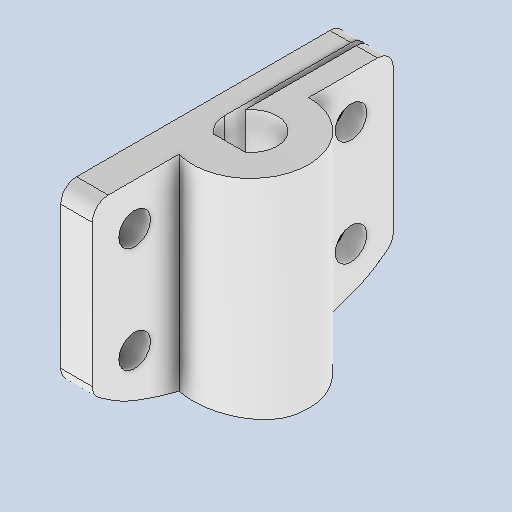
# Autodesk Inventor part: eixo_motor
Saved by Autodesk Inventor 2023.2 (Build 272271000, 271)
## iProperties
Created: 2023-04-13
Part Number: eixo_motor
Material: ABS plástico
Document SubType Name: Modeling
Designer: Edilson
Density: 1.06 g/cm^3
Appearance: Suave - Branco
Author: Edilson
Autodesk Inventor part; units mm, degrees
ref_plane "YZ Plane" through (0, 0, 0) normal (1, 0, 0) x (0, 1, 0)
ref_plane "XZ Plane" through (0, 0, 0) normal (0, 1, 0) x (-1, 0, 0)
sketch "Esboço5" plane through (0, 0, 0) normal (0, 1, 0) x (-1, 0, 0)
  line L0 (-13.5, 0) -> (-13.5, -1)
  line L1 (-13.5, -1) -> (0, -1)
  line L2 (13.5, -1) -> (13.5, 0)
  arc A0 (-5.5, -3.5) -> (5.2915, -2) centre (0, -3.5) ccw
  line L3 (2, -3.5) -> (2, -2)
  line L4 (2, -3.5) -> (2, -5)
  line L5 (-13.5, -1.5) -> (-1.5, -1.5)
  line L6 (-13.5, -1.5) -> (-13.5, -3.5)
  line L7 (-13.5, -3.5) -> (-5.5, -3.5)
  line L8 (13.5, -1) -> (13.5, -2)
  line L9 (13.5, -2) -> (5.2915, -2)
  arc A1 (2, -2) -> (0, -1) centre (0, -3.5) ccw
  arc A2 (-1.5, -1.5) -> (2, -5) centre (0, -3.5) ccw
  line L10 (13.5, 0) -> (13.5, 1)
  line L11 (13.5, 0) -> (14.5, 0) construction
  line L12 (13.5, 1) -> (-13.5, 1)
  line L13 (-13.5, 1) -> (-13.5, 0)
  constraints: 28 end point, 6 perpendicular, 6 point on circle, 3 centre point, 1 horizontal, 1 parallel, 1 point on line, 1 vertical
extrude "Extrusão4" add sketch "Esboço5" against normal blind 20
sketch "Esboço6" plane through (-5.2915, 0, -2) normal (0, 0, -1) x (-1, 0, 0)
  circle A0 centre (4.2085, -16) radius 1.5
  circle A1 centre (4.2085, -6) radius 1.5
  line L0 (8.2085, -20) -> (0, -20) projected
  line L1 (8.2085, 0) -> (8.2085, -20) projected
  point P0 (-5.2915, 0)
  point P1 (4.1042, -20)
  dimension "d51" = 3
  dimension "d52" = 3
  dimension "d53" = 4
  dimension "d54" = 4
  dimension "d55" = 10
  dimension "d56" = 4
  constraints: 2 centre point, 1 midpoint
  measures "d51" diameter of A0
  measures "d52" diameter of A1
  measures "d53" vertical distance of point (4.104, -20) A0.centre
  measures "d54" distance from line of L1 A0.centre
  measures "d55" distance of A1.centre A0.centre
  measures "d56" distance from line of L1 A1.centre
extrude "Extrusão5" cut sketch "Esboço6" against normal through all
sketch "Esboço7" plane through (13.5, 0, -3.5) normal (0, 0, -1) x (-1, 0, 0)
  circle A0 centre (4, -16) radius 1.5
  circle A1 centre (4, -6) radius 1.5
  line L0 (8, -20) -> (0, -20) projected
  line L1 (0, 0) -> (0, -20) projected
  point P0 (13.5, 0)
  point P1 (4, -20)
  dimension "d59" = 3
  dimension "d60" = 3
  dimension "d61" = 4
  dimension "d62" = 4
  dimension "d63" = 4
  dimension "d64" = 10
  constraints: 2 centre point, 1 midpoint
  measures "d59" diameter of A0
  measures "d60" diameter of A1
  measures "d61" distance of point (4, -20) A0.centre
  measures "d62" distance from line of L1 A0.centre
  measures "d63" distance from line of L1 A1.centre
  measures "d64" distance of A1.centre A0.centre
extrude "Extrusão6" cut sketch "Esboço7" against normal through all
ref_plane "Plano de trabalho2" through (-12, 0, 1) normal (0, 0, 1) x (1, 0, 0)
sketch "Esboço9" plane through (-12, 0, 1) normal (0, 0, 1) x (1, 0, 0)
  spline S0 degree 3 poles (57.7409, -54.8608) (52.9733, -36.0784) (42.5201, -20.9336) (27.3088, -10.4014) knots 0 0 0 0 1 1 1 1
  line L0 (57.7409, -54.8608) -> (52.9733, -36.0784) construction
  line L1 (52.9733, -36.0784) -> (42.5201, -20.9336) construction
  line L2 (42.5201, -20.9336) -> (27.3088, -10.4014) construction
  line L3 (27.3088, -10.4014) -> (21.7838, -6.5759)
  spline S1 degree 3 poles (21.7838, -6.5759) (20.7493, -5.8596) (20.3116, -5.8348) (19.1032, -5.4031) knots 0 0 0 0 1 1 1 1
  line L4 (21.7838, -6.5759) -> (20.7493, -5.8596) construction
  line L5 (20.7493, -5.8596) -> (20.3116, -5.8348) construction
  line L6 (20.3116, -5.8348) -> (19.1032, -5.4031) construction
  spline S2 degree 3 poles (19.1032, -5.4031) (17.5273, -4.8402) (15.1033, -4.0535) (11.9998, -4.064) knots 0 0 0 0 1 1 1 1
  line L7 (19.1032, -5.4031) -> (17.5273, -4.8402) construction
  line L8 (17.5273, -4.8402) -> (15.1033, -4.0535) construction
  line L9 (15.1033, -4.0535) -> (11.9998, -4.064) construction
  spline S3 degree 3 poles (11.9998, -4.064) (8.8963, -4.0535) (6.4726, -4.8398) (4.8965, -5.4032) knots 0 0 0 0 1 1 1 1
  line L10 (11.9998, -4.064) -> (8.8963, -4.0535) construction
  line L11 (8.8963, -4.0535) -> (6.4726, -4.8398) construction
  line L12 (6.4726, -4.8398) -> (4.8965, -5.4032) construction
  spline S4 degree 3 poles (4.8965, -5.4032) (3.6877, -5.8353) (3.3099, -5.9475) (2.2535, -6.6648) knots 0 0 0 0 1 1 1 1
  line L13 (4.8965, -5.4032) -> (3.6877, -5.8353) construction
  line L14 (3.6877, -5.8353) -> (3.3099, -5.9475) construction
  line L15 (3.3099, -5.9475) -> (2.2535, -6.6648) construction
  line L16 (2.2535, -6.6648) -> (-3.3045, -10.439)
  spline S5 degree 3 poles (-3.3045, -10.439) (-18.597, -20.8233) (-28.9756, -36.0782) (-33.7434, -54.8605) knots 0 0 0 0 1 1 1 1
  line L17 (-3.3045, -10.439) -> (-18.597, -20.8233) construction
  line L18 (-18.597, -20.8233) -> (-28.9756, -36.0782) construction
  line L19 (-28.9756, -36.0782) -> (-33.7434, -54.8605) construction
  ellipse E0 centre (-9.9997, -23.559) end of major axis (-9.9997, -25.1466) minor radius 1.5876
  ellipse E1 centre (34, -23.559) end of major axis (34, -25.1466) minor radius 1.5876
  ellipse E2 centre (-9.9997, -23.559) end of major axis (-9.9997, -26.759) minor radius 3.2
  spline S6 degree 3 poles (55.5624, -55.1832) (51.0219, -37.2964) (40.7593, -23.2973) (26.5685, -12.7553) knots 0 0 0 0 1 1 1 1
  line L20 (55.5624, -55.1832) -> (51.0219, -37.2964) construction
  line L21 (51.0219, -37.2964) -> (40.7593, -23.2973) construction
  line L22 (40.7593, -23.2973) -> (26.5685, -12.7553) construction
  line L23 (26.5685, -12.7553) -> (21.337, -9.203)
  spline S7 degree 3 poles (21.337, -9.203) (20.3311, -8.5199) (19.9165, -8.4914) (18.7657, -8.0804) knots 0 0 0 0 1 1 1 1
  line L24 (21.337, -9.203) -> (20.3311, -8.5199) construction
  line L25 (20.3311, -8.5199) -> (19.9165, -8.4914) construction
  line L26 (19.9165, -8.4914) -> (18.7657, -8.0804) construction
  spline S8 degree 3 poles (18.7657, -8.0804) (17.2648, -7.5442) (14.9553, -6.7946) (11.9998, -6.8046) knots 0 0 0 0 1 1 1 1
  line L27 (18.7657, -8.0804) -> (17.2648, -7.5442) construction
  line L28 (17.2648, -7.5442) -> (14.9553, -6.7946) construction
  line L29 (14.9553, -6.7946) -> (11.9998, -6.8046) construction
  spline S9 degree 3 poles (11.9998, -6.8046) (9.0442, -6.7946) (6.7347, -7.5442) (5.2338, -8.0804) knots 0 0 0 0 1 1 1 1
  line L30 (11.9998, -6.8046) -> (9.0442, -6.7946) construction
  line L31 (9.0442, -6.7946) -> (6.7347, -7.5442) construction
  line L32 (6.7347, -7.5442) -> (5.2338, -8.0804) construction
  spline S10 degree 3 poles (5.2338, -8.0804) (4.083, -8.4914) (3.6685, -8.5199) (2.6625, -9.203) knots 0 0 0 0 1 1 1 1
  line L33 (5.2338, -8.0804) -> (4.083, -8.4914) construction
  line L34 (4.083, -8.4914) -> (3.6685, -8.5199) construction
  line L35 (3.6685, -8.5199) -> (2.6625, -9.203) construction
  line L36 (2.6625, -9.203) -> (-2.5689, -12.7553)
  spline S11 degree 3 poles (-2.5689, -12.7553) (-16.7598, -23.2973) (-27.0223, -37.2964) (-31.5628, -55.1832) knots 0 0 0 0 1 1 1 1
  line L37 (-2.5689, -12.7553) -> (-16.7598, -23.2973) construction
  line L38 (-16.7598, -23.2973) -> (-27.0223, -37.2964) construction
  line L39 (-27.0223, -37.2964) -> (-31.5628, -55.1832) construction
  ellipse E3 centre (34, -23.559) end of major axis (34, -26.759) minor radius 3.2
  circle A0 centre (21.5, -16) radius 1.5
  circle A1 centre (21.5, -16) radius 1.5
  circle A2 centre (34, -23.559) radius 1.5
  line L40 (24.1257, -3.1935) -> (25.5, -4.1451)
  line L41 (-1.5, -4.2408) -> (-0.0576, -3.2613)
  line L42 (25.5, -1.5) -> (25.5, -18.5)
  line L43 (25.5, -4.1451) -> (25.5, 0)
  line L44 (25.5, 0) -> (-1.5, 0)
  line L45 (-1.5, 0) -> (-1.5, -4.2408)
  line L46 (-1.5, -1.5) -> (-1.5, -18.5)
  spline S12 degree 4 poles (-0.0576, -3.2613) (0.3901, -2.9579) (0.8455, -2.665) (1.7229, -2.1882) (2.6538, -1.8305) (3.0838, -1.683) (3.5118, -1.5292) knots 0 0 0 0 0 0.543292 0.543292 1 1 1 1 1
  spline S13 degree 4 poles (3.5118, -1.5292) (4.3634, -1.2239) (5.2232, -0.9408) (6.9422, -0.4668) (8.699, -0.163) (9.5701, -0.0586) (10.4443, 0) knots 0 0 0 0 0 0.508027 0.508027 1 1 1 1 1
  spline S14 degree 4 poles (13.5551, 0) (14.4294, -0.0586) (15.3006, -0.163) (17.0573, -0.4669) (18.7762, -0.9409) (19.6358, -1.2238) (20.4873, -1.5289) knots 0 0 0 0 0 0.49206 0.49206 1 1 1 1 1
  spline S15 degree 4 poles (20.4871, -1.5289) (20.8593, -1.6632) (21.2378, -1.7784) (22.1946, -2.0885) (23.1045, -2.5256) (23.6246, -2.8472) (24.1257, -3.1935) knots 0 0 0 0 0 0.393579 0.393579 1 1 1 1 1
  point P0 (12, 0)
  dimension "d69" = 3
  dimension "d70" = 3
  dimension "d71" = 7.559
  dimension "d72" = 12.5
  dimension "d73" = 4.114
  dimension "d74" = 27
  constraints: 18 end point, 4 point on line, 2 centre point, 1 coincident, 1 perpendicular, 1 vertical, 56 other
  measures "d69" diameter of A1
  measures "d70" diameter of A2
  measures "d71" vertical distance of A1.centre A2.centre
  measures "d72" horizontal distance of A0.centre A2.centre
  measures "d73" distance between parallel lines of L3 L40
  measures "d74" distance of L43.end L44.end
extrude "Extrusão7" cut sketch "Esboço9" against normal through all contours L40 S15 S14 L44 L43 L42 | S13 S12 L41 L45 L44
fillet "Arredondamento2" radius 1.5 6 edges at (-13.5, -20, -0.5) (13.5, -20, 0) (13.5, -20, -2.5) (13.5, -4.1451, -2.5) (13.5, -4.1451, 0) (-13.5, -4.2408, -0.5)
